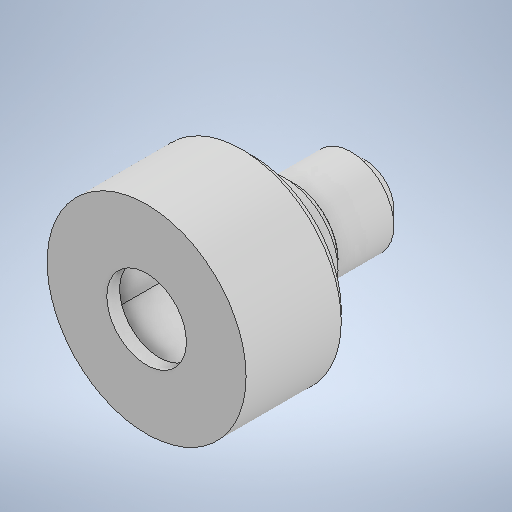
# Autodesk Inventor part: Shaft_to_beam_interface
Saved by Autodesk Inventor 2025.1 (Build 291241000, 241)
## iProperties
Created: 2025-05-22
Part Number: Shaft_to_beam_interface
Material: Generic
Document SubType Name: Modeling
Designer: Andreas' PC
Density: 1 g/cm^3
Appearance: Default
Author: Andreas' PC
## iProperties of the stored document Shaft_to_beam_interface_3DPrint.ipt
Created: 2025-05-22
Part Number: Shaft_to_beam_interface_3DPrint
Material: Generic
Document SubType Name: Modeling
Designer: Andreas' PC
Density: 1 g/cm^3
Appearance: Default
Author: Andreas' PC
Autodesk Inventor part; units mm, degrees
ref_plane "YZ Plane" through (0, 0, 0) normal (1, 0, 0) x (0, 1, 0)
ref_plane "XZ Plane" through (0, 0, 0) normal (0, 1, 0) x (-1, 0, 0)
ref_plane "XY Plane" through (0, 0, 0) normal (0, 0, 1) x (1, 0, 0)
sketch "Sketch1" plane through (0, 0, 0) normal (0, 0, 1) x (1, 0, 0)
  circle A0 centre (0, 0) radius 3
  dimension "d0" = 6
  constraints: 1 centre point, 1 coincident
  measures "d0" diameter of A0
extrude "Extrusion1" add sketch "Sketch1" along normal blind 5
sketch "Sketch2" plane through (0, 0, 5) normal (0, 0, 1) x (1, 0, 0)
  circle A0 centre (0, 0) radius 3.775
  dimension "d3" = 7.55
  constraints: 1 centre point, 1 coincident
  measures "d3" diameter of A0
extrude "Extrusion2" add sketch "Sketch2" along normal blind 3
sketch "Sketch3" plane through (0, 0, 8) normal (0, 0, 1) x (1, 0, 0)
  circle A0 centre (0, 0) radius 7
  circle A1 centre (0, 0) radius 2.8
  dimension "d7" = 14
  dimension "d25" = 5.6
  constraints: 3 coincident, 2 centre point
  measures "d7" diameter of A0
  measures "d25" diameter of A1
extrude "Extrusion3" add sketch "Sketch3" along normal blind 2.2
sketch "Sketch5" plane through (0, 0, 10.2) normal (0, 0, 1) x (1, 0, 0)
  line L0 (-4.15, 2.396) -> (0, 4.792)
  line L1 (0, 4.792) -> (4.15, 2.396)
  line L2 (4.15, 2.396) -> (4.15, -2.396)
  line L3 (4.15, -2.396) -> (0, -4.792)
  line L4 (0, -4.792) -> (-4.15, -2.396)
  line L5 (-4.15, -2.396) -> (-4.15, 2.396)
  circle A0 centre (0, 0) radius 7
  dimension "d19" = 8.3
  constraints: 12 end point, 2 coincident, 1 centre point, 13 other
  measures "d19" distance between parallel lines of L2 L5
extrude "Extrusion5" add sketch "Sketch5" along normal blind 4.3
sketch "Sketch6" plane through (0, 0, 14.5) normal (0, 0, 1) x (1, 0, 0)
  circle A0 centre (0, 0) radius 7
  circle A1 centre (0, 0) radius 2.8
  dimension "d24" = 5.6
  constraints: 2 centre point, 2 coincident
  measures "d24" diameter of A1
extrude "Extrusion6" add sketch "Sketch6" along normal blind 0.9
chamfer "Chamfer1" distance 1 angle 45 1 edges at (-3, 0, 0)
chamfer "Chamfer2" distance 0.7 angle 45 2 edges at (-3.775, 0, 5) (-7, 0, 8)
equation "\"m3_hex_s\" = 5.4"
equation "\"m3_hex_m\" = 2.3"
equation "\"m3_rund_d\" = 5.95"
equation "\"m3_rund_m\" = 2.6"
equation "\"l______________l\" = 0"
equation "\"Lengths\" = 0"
equation "\"L20\" = 0"
equation "\"L25\" = 0"
equation "\"L16\" = 0"
equation "\"L12\" = 0"
equation "\"L8\" = 0"
equation "\"L4\" = 0"
equation "\"m3_s\" = 5.4"
equation "\"m3_m\" = 2.3"
body "Solid1"
